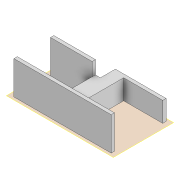
# Autodesk Inventor part: Odometry holder for metal drive train
Saved by Autodesk Inventor 2020 (Build 240168000, 168)
## iProperties
Created: 2020-03-04
Part Number: Odometry holder for metal drive train
Material: Generic
Document SubType Name: Modeling
Designer: ball
Density: 1 g/cm^3
Appearance: Default
Author: ball
Autodesk Inventor part; units mm, degrees
ref_plane "YZ Plane" through (0, 0, 0) normal (1, 0, 0) x (0, 1, 0)
ref_plane "XY Plane" through (0, 0, 0) normal (0, 0, 1) x (1, 0, 0)
sketch "Sketch1" plane through (0, 0, 0) normal (0, 1, 0) x (-1, 0, 0)
  line L0 (10.16, 20.955) -> (-64.135, 20.955)
  line L1 (-64.135, 20.955) -> (-64.135, 18.415)
  line L2 (-64.135, 18.415) -> (10.16, 18.415)
  line L3 (10.16, 18.415) -> (10.16, 20.955)
  line L4 (10.16, -6.985) -> (-21.59, -6.985)
  line L5 (-21.59, -6.985) -> (-21.59, -9.525)
  line L6 (-21.59, -9.525) -> (10.16, -9.525)
  line L7 (10.16, -9.525) -> (10.16, -6.985)
  point P0 (0, 0)
  dimension "d0" = 74.295
  dimension "d1" = 2.54
  dimension "d2" = 10.16
  dimension "d3" = 20.955
  dimension "d4" = 31.75
  dimension "d5" = 2.54
  dimension "d6" = 10.16
  dimension "d7" = 30.48
  constraints: 16 end point, 4 parallel, 2 horizontal, 2 perpendicular
  measures "d0" distance of L2.end L1.end
  measures "d1" distance of L1.end L0.end
  measures "d2" distance from line of L3 point (0, 0)
  measures "d3" distance from line of L0 point (0, 0)
  measures "d4" distance of L6.end L5.end
  measures "d5" distance of L5.end L4.end
  measures "d6" distance from line of L7 point (0, 0)
  measures "d7" distance between parallel lines of L6 L0
extrude "Extrusion1" add sketch "Sketch1" along normal blind 25.4
sketch "Sketch2" plane through (0, 0, 0) normal (0, 1, 0) x (-1, 0, 0)
  line L0 (-64.135, 18.415) -> (10.16, 18.415) projected
  line L1 (10.16, -6.985) -> (-21.59, -6.985) projected
  line L2 (-21.59, 18.415) -> (-34.29, 18.415)
  line L3 (10.16, 18.415) -> (10.16, 20.955) projected
  line L4 (-21.59, -9.525) -> (-25.4, -9.525)
  line L5 (-21.59, -6.985) -> (-21.59, -9.525) projected
  line L6 (-21.59, -9.525) -> (-21.59, 18.415)
  line L7 (-25.4, -9.525) -> (-25.4, -20.955)
  line L8 (-25.4, -20.955) -> (-34.29, -20.955)
  line L9 (-34.29, -20.955) -> (-34.29, 18.415)
  line L10 (-64.135, 18.415) -> (10.16, 18.415) projected
  line L11 (10.16, -9.525) -> (10.16, -6.985) projected
  line L12 (10.16, 20.955) -> (-64.135, 20.955) projected
  point P0 (0, 0)
  point P1 (-21.59, -6.985)
  dimension "d16" = 35.56
  dimension "d17" = 41.91
  dimension "d18" = 12.7
  constraints: 12 end point, 1 collinear, 1 horizontal, 1 perpendicular, 1 point on line, 1 vertical
  measures "d16" distance between parallel lines of L7 L11
  measures "d17" distance between parallel lines of L8 L12
  measures "d18" distance between parallel lines of L9 L6
extrude "Extrusion2" add sketch "Sketch2" along normal blind 15.24
sketch "Sketch4" plane through (0, 0, 0) normal (0, 1, 0) x (-1, 0, 0)
  line L0 (-34.29, -20.955) -> (-25.4, -20.955) projected
  line L1 (-34.29, -20.955) -> (-64.135, -20.955)
  line L2 (-64.135, -20.955) -> (-64.135, -18.415)
  line L3 (-64.135, -18.415) -> (-34.29, -18.415)
  line L4 (-34.29, -18.415) -> (-34.29, -20.955)
  point P0 (0, 0)
  dimension "d19" = 29.845
  dimension "d20" = 2.54
  constraints: 8 end point, 2 parallel, 1 horizontal, 1 perpendicular
  measures "d19" distance of L2.end L3.end
  measures "d20" distance of L1.end L2.end
extrude "Extrusion3" add sketch "Sketch4" along normal blind 15.24
equation "\"d5\" = d1"
equation "\"d6\" = d2"
body "Solid1"
